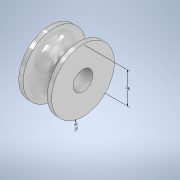
# Autodesk Inventor part: wheel
Saved by Autodesk Inventor 2022 (Build 260153000, 153)
## iProperties
Created: 2022-10-27
Part Number: wheel
Material: Generic
Document SubType Name: Modeling
Designer: matia
Density: 1 g/cm^3
Appearance: Default
Author: matia
Autodesk Inventor part; units mm, degrees
ref_plane "YZ Plane" through (0, 0, 0) normal (1, 0, 0) x (0, 1, 0)
ref_plane "XZ Plane" through (0, 0, 0) normal (0, 1, 0) x (-1, 0, 0)
ref_plane "XY Plane" through (0, 0, 0) normal (0, 0, 1) x (1, 0, 0)
sketch "Sketch1" plane through (0, 0, 0) normal (0, 0, 1) x (1, 0, 0)
  line L0 (0, 0) -> (0, 9.1966)
  arc A0 (-3.556, 9.1966) -> (3.556, 9.1966) centre (0, 9.1966) ccw
  line L1 (-3.556, 9.1966) -> (-3.556, 1.5328)
  line L2 (3.556, 1.5328) -> (3.556, 9.1966)
  line L3 (-3.556, 1.5328) -> (3.556, 1.5328)
  line L4 (-3.556, 1.5328) -> (-4.826, 1.5328)
  line L5 (-4.826, 1.5328) -> (3.556, 1.5328)
  line L6 (3.556, 1.5328) -> (4.826, 1.5328)
  line L7 (4.826, 1.5328) -> (4.826, 9.1966)
  line L8 (4.826, 9.1966) -> (3.556, 9.1966)
  line L9 (-3.556, 9.1966) -> (-4.826, 9.1966)
  line L10 (-4.826, 9.1966) -> (-4.826, 1.5328)
  line L11 (-8.7255, 0) -> (10.8498, 0)
  constraints: 24 end point, 4 perpendicular, 3 horizontal, 2 point on circle, 2 vertical, 1 centre point, 1 coincident, 1 collinear, 1 point on line, 1 tangent
revolve "Revolution1" add sketch "Sketch1" angle 360 about axis through (-8.7255, 0, 0) along (1, 0, 0)
sketch "Sketch2" plane through (4.826, 0, 0) normal (1, 0, 0) x (0, 0, -1)
  circle A0 centre (0, 0) radius 2.8575
  dimension "d10" = 5.715
  constraints: 1 centre point, 1 coincident
  measures "d10" diameter of A0
extrude "Extrusion1" cut sketch "Sketch2" against normal through all
body "Solid1"
